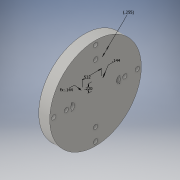
# Autodesk Inventor part: Part1
Saved by Autodesk Inventor 2016 (Build 200138000, 138)
## iProperties
Created: 2017-09-28
Part Number: Part1
Material: Generic
Document SubType Name: Modeling
Designer: Student
Density: 1 g/cm^3
Appearance: Default
Author: Student
Autodesk Inventor part; units mm, degrees
ref_plane "YZ Plane" through (0, 0, 0) normal (1, 0, 0) x (0, 1, 0)
ref_plane "XZ Plane" through (0, 0, 0) normal (0, 1, 0) x (-1, 0, 0)
ref_plane "XY Plane" through (0, 0, 0) normal (0, 0, 1) x (1, 0, 0)
sketch "Sketch1" plane through (0, 0, 0) normal (0, 1, 0) x (-1, 0, 0)
  line L0 (0, 0) -> (0, -31.748)
  line L1 (0, -31.748) -> (7.62, -31.748)
  line L2 (7.62, -31.748) -> (7.62, -26.16)
  line L3 (7.62, -26.16) -> (4.953, -26.16)
  line L4 (4.953, -26.16) -> (4.953, -23.493)
  line L5 (4.953, -23.493) -> (7.62, -23.493)
  line L6 (7.62, -23.493) -> (7.62, -17.016)
  line L7 (7.62, -17.016) -> (2.54, -17.016)
  line L8 (2.54, -17.016) -> (2.54, 0)
  line L9 (0, 0) -> (2.54, 0)
  dimension "d0" = 31.748
  dimension "d1" = 7.62
  dimension "d2" = 5.588
  dimension "d3" = 2.667
  dimension "d4" = 2.667
  dimension "d5" = 6.477
  dimension "d6" = 5.08
  dimension "d7" = 2.54
  constraints: 20 end point, 5 horizontal, 5 vertical
  measures "d0" distance of L0.start L0.end
  measures "d1" distance of L0.end L1.end
  measures "d2" distance of L1.end L2.end
  measures "d3" distance of L2.end L3.end
  measures "d4" distance of L3.end L4.end
  measures "d5" distance of L5.end L6.end
  measures "d6" distance of L6.end L7.end
  measures "d7" distance of L0.start L8.end
revolve "Revolution1" add sketch "Sketch1" angle 360 about axis through (0, 0, 0) along (-1, 0, 0)
sketch "Sketch2" plane through (-7.62, 0, 0) normal (-1, 0, 0) x (0, 0, 1)
  circle A0 centre (28.954, 0) radius 1.5
  circle A1 centre (0, 0) radius 31.748 projected
  line L0 (31.748, 0) -> (26.16, 0)
  circle A2 centre (0, 0) radius 26.16 projected
  circle A3 centre (0, 28.954) radius 1.5
  circle A4 centre (-28.954, 0) radius 1.5
  circle A5 centre (0, -28.954) radius 1.5
  dimension "d9" = 3
  dimension "d12" = 360
  constraints: 4 centre point, 2 end point, 2 horizontal alignment, 1 coincident, 1 horizontal, 1 midpoint, 11 other
  measures "d9" diameter of A0
extrude "Extrusion1" cut sketch "Sketch2" against normal blind 12.7 contours L0 A0 | A0 L0 | A3 | A4 | A5
sketch "Sketch3" plane through (0, 0, 0) normal (1, 0, 0) x (0, 0, -1)
  circle A0 centre (0, 0) radius 23.493 projected
  circle A1 centre (0, 0) radius 20.2545
  circle A2 centre (20.2545, 0) radius 1.5
  circle A3 centre (0, 20.2545) radius 1.5
  circle A4 centre (-20.2545, 0) radius 1.5
  circle A5 centre (0, -20.2545) radius 1.5
  dimension "d17" = 3.2385
  dimension "d18" = 3
  dimension "d21" = 360
  constraints: 4 centre point, 1 coincident, 1 horizontal alignment, 11 other
  measures "d18" diameter of A2
sketch "Sketch4" plane through (-7.62, 0, 0) normal (-1, 0, 0) x (0, 0, 1)
  circle A0 centre (0, 0) radius 17.016 projected
  circle A1 centre (0, 0) radius 23.493 projected
  dimension "d16" = 6.477
  measures "d16" radial gap between concentric circles of A0 A1
extrude "Extrusion2" cut sketch "Sketch3" against normal blind 5.08 contours A1 A2 | A1 A2 | A3 A1 | A1 A3 | A5 A1 | A1 A5 | A4 A1 | A1 A4
sketch "Sketch5" plane through (-2.54, 0, 0) normal (-1, 0, 0) x (0, 0, 1)
  circle A0 centre (0, 0) radius 17.016 projected
  line L0 (-17.016, 0) -> (17.016, 0)
  line L1 (-14.478, -9.9949) -> (14.478, -9.9949)
  line L2 (-14.478, 9.9949) -> (14.478, 9.9949)
  line L3 (14.478, 9.9949) -> (14.478, -9.9949)
  line L4 (-14.478, 9.9949) -> (-14.478, -9.9949)
  arc A1 (16.8267, -2.5309) -> (16.8267, 2.5309) centre (0, 0) ccw
  point P0 (0, 9.9949)
  point P1 (14.478, 0)
  dimension "d25" = 28.956
  dimension "d26" = 19.9898
  constraints: 10 end point, 6 point on circle, 3 horizontal, 3 midpoint, 2 vertical, 1 centre point, 1 horizontal alignment, 1 vertical alignment
  measures "d25" distance of L2.start L2.end
  measures "d26" distance of L2.end L1.end
sketch "Sketch6" plane through (-7.62, 0, 0) normal (-1, 0, 0) x (0, 0, 1)
  circle A0 centre (0, 0) radius 17.016 projected
  circle A1 centre (17.016, 0) radius 2.54
  arc A2 (16.8264, -2.5329) -> (16.8264, 2.5329) centre (0, 0) ccw
  circle A3 centre (-17.016, -0.0173) radius 2.54
  arc A4 (-16.829, 2.5158) -> (-16.8238, -2.55) centre (0, 0) ccw
  dimension "d27" = 5.08
  dimension "d28" = 5.08
  constraints: 16 point on circle, 4 centre point
  measures "d27" diameter of A1
  measures "d28" diameter of A3
extrude "Extrusion3" cut sketch "Sketch6" against normal blind 12.7 contours A0 A1 | A3 A0 picked at (16.1885, -0.4913) picked at (-16.1553, -0.0173)
sketch "Sketch7" plane through (-2.54, 0, 17.016) normal (-1, 0, 0) x (0, 0, 1)
  circle A0 centre (-25.6012, 5.588) radius 1.8288
  circle A1 centre (-8.4308, 5.588) radius 1.8288
  arc A2 (-33.8398, -2.55) -> (-33.8449, 2.5158) centre (-34.0319, -0.0173) ccw projected
  line L0 (-31.4919, -0.0173) -> (-2.4894, -0.0173) construction
  line L1 (-25.6012, 5.588) -> (-8.4308, 5.588)
  circle A3 centre (-25.6012, 5.588) radius 1.8288
  circle A4 centre (-8.4308, 5.588) radius 1.8288
  point P0 (-17.016, 0)
  point P1 (-17.016, 5.588)
  dimension "d31" = 3.6576
  dimension "d32" = 3.6576
  dimension "d33" = 13.5128
  dimension "d34" = 5.588
  constraints: 4 centre point, 4 end point, 2 coincident, 2 concentric, 2 horizontal, 1 midpoint, 1 point on circle, 1 vertical alignment
  measures "d31" diameter of A0
  measures "d32" diameter of A1
  measures "d34" distance of point (-17.016, 5.588) point (-17.016, 0)
equation "\"d28\" = d27"
equation "\"d32\" = d31"
body "Solid1"
